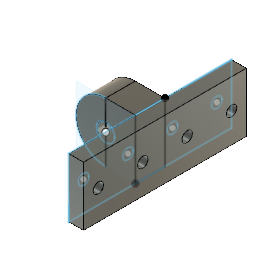
camera_joint_male (Autodesk Fusion 360 design; units mm, degrees)
Autodesk Fusion 360 part; units mm, degrees
note: some values were not read from the file. Chosen so that the rebuilt part matches the saved one: that a step has no effect. Set by a fixed rule: which sketch regions a step uses.
ref_plane "WorkPlane1" through (-98.2453, -42.8288, 162.8804) normal (-0.999826, -0.005173, -0.017916) x (-0.018434, 0.129368, 0.991425)
pattern_linear "R-Pattern1" [no effect]
extrude "Extrude9" [no effect]
extrude "Extrude10" [no effect]
sketch "Sketch12" plane through (-95.5151, -0.4942, -1.7115) normal (-0.999826, -0.005173, -0.017916) x (0.005174, -0.999987, 0)
sketch "Sketch13" plane through (0.6338, -122.4984, 0) normal (0.005174, -0.999987, 0) x (0.999987, 0.005174, 0)
extrude "Extrude15" [no effect]
sketch "Sketch16" plane through (0, 0, 0) normal (1, 0, 0) x (0, 1, 0)
  line L0 (10, 50) -> (65, 50)
  line L1 (65, 50) -> (65, 30)
  line L2 (65, 30) -> (10, 30)
  line L3 (10, 30) -> (10, 50)
  circle A0 centre (45, 40) radius 1.75
  circle A1 centre (60, 40) radius 1.75
  circle A2 centre (30, 40) radius 1.75
  circle A3 centre (15, 40) radius 1.75
  dimension "d55" = 55
  dimension "d56" = 20
  dimension "d60" = 3.5
  dimension "d61" = 3.5
  dimension "d62" = 15
  dimension "d63" = 3.5
  dimension "d64" = 3.5
  dimension "d66" = 15
  dimension "d67" = 5
  dimension "d68" = 15
  dimension "d69" = 10
  constraint horizontal L0
  constraint vertical L1
  constraint horizontal L2
  constraint vertical L3
  constraint horizontal A2.centre A3.centre
  measures "d55" distance of L0.start L0.end
  measures "d56" distance of L0.end L1.end
  measures "d60" diameter of A1
  measures "d61" diameter of A0
  measures "d62" distance of A1.centre A0.centre
  measures "d63" diameter of A3
  measures "d64" diameter of A2
  measures "d66" horizontal distance of A2.centre A3.centre
  measures "d67" distance of L1 A1.centre
  measures "d68" distance of A0.centre A2.centre
  measures "d69" distance of L0 A1.centre
extrude "Extrude16" add sketch "Sketch16" along normal blind 5
sketch "Sketch17" plane through (0, 0, 0) normal (-1, 0, 0) x (0, -1, 0)
  circle A0 centre (-45, 40) radius 1.75
  circle A1 centre (-30, 40) radius 1.75
  circle A2 centre (-15, 40) radius 1.75
  circle A3 centre (-60, 40) radius 1.75
  line L0 (-65, 30) -> (-10, 30)
  line L1 (-10, 30) -> (-10, 50)
  line L2 (-10, 50) -> (-65, 50)
  line L3 (-65, 50) -> (-65, 30)
  line L4 (-42.5, 50) -> (-32.5, 50)
  line L5 (-32.5, 50) -> (-32.5, 30)
  line L6 (-32.5, 30) -> (-42.5, 30)
  line L7 (-42.5, 30) -> (-42.5, 50)
  dimension "d72" = 10
  dimension "d73" = 2.5
  constraint horizontal L4
  constraint vertical L5
  constraint horizontal L6
  constraint vertical L7
  constraint coincident L0 L5.end
  constraint coincident L2 L4.start
  measures "d72" distance of L4.start L4.end
  measures "d73" horizontal distance of A0.centre L4.start
extrude "Extrude17" add sketch "Sketch17" along normal blind 20 contours L0 L2 L4 L5 L6 L7
sketch "Sketch18" plane through (0, 32.5, 0) normal (0, -1, 0) x (1, 0, 0)
  line L0 (0, 30) -> (0, 50)
  line L1 (0, 50) -> (-20, 50)
  line L2 (-20, 50) -> (-20, 30)
  line L3 (-20, 30) -> (0, 30)
  line L4 (-10, 50) -> (-10, 30)
  arc A0 (-10, 50) -> (-20, 40) centre (-10, 40) ccw
  arc A1 (-20, 40) -> (-10, 30) centre (-10, 40) ccw
  circle A2 centre (-10, 40) radius 3
  dimension "d76" = 10
  dimension "d77" = 10
  dimension "d78" = 6
  constraint vertical L4
  constraint midpoint L3 L4.end
  constraint coincident L4.start A0.start
  constraint coincident A0.end A1.start
  constraint coincident L4.end A1.end
  constraint concentric A1 A2
  measures "d76" radius of A0
  measures "d77" radius of A1
  measures "d78" diameter of A2
extrude "Extrude18" cut sketch "Sketch18" against normal blind 10 contours L2 L3 A1 | L1 L2 A0 | L4 A2 | L4 A2
